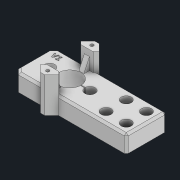
# Autodesk Inventor part: z-top
Saved by Autodesk Inventor 2021 (Build 250183000, 183)
## iProperties
Created: 2021-06-08
Part Number: z-top
Material: Generic
Document SubType Name: Modeling
Designer: arbra
Density: 1 g/cm^3
Appearance: Default
Author: arbra
Autodesk Inventor part; units mm, degrees
ref_plane "YZ Plane" through (0, 0, 0) normal (1, 0, 0) x (0, 1, 0)
ref_plane "XZ Plane" through (0, 0, 0) normal (0, 1, 0) x (-1, 0, 0)
ref_plane "XY Plane" through (0, 0, 0) normal (0, 0, 1) x (1, 0, 0)
sketch "Sketch1" plane through (0, 0, 0) normal (0, 1, 0) x (-1, 0, 0)
  line L0 (0, -40.5879) -> (0, 40.5879) construction
  line L1 (-98.4, 0) -> (58.4, 0) construction
  circle A0 centre (0, 0) radius 5
  arc A1 (14.9389, -0.375) -> (14.9389, 0.375) centre (20, 0) ccw
  line L2 (14.9389, -0.375) -> (8.9389, -0.375)
  line L3 (8.9389, -0.375) -> (8.9389, 0.375)
  line L4 (8.9389, 0.375) -> (14.9389, 0.375)
  line L5 (20, 0) -> (8.9389, 0) construction
  arc A2 (-14.9389, 0.375) -> (-14.9389, -0.375) centre (-20, 0) ccw
  line L6 (-14.9389, -0.375) -> (-8.9389, -0.375)
  line L7 (-8.9389, -0.375) -> (-8.9389, 0.375)
  line L8 (-8.9389, 0.375) -> (-14.9389, 0.375)
  line L9 (-36, 20) -> (-76, 20) construction
  line L10 (-76, 20) -> (-76, -20)
  line L11 (-76, -20) -> (-36, -20) construction
  line L12 (-36, -20) -> (-36, 20) construction
  line L13 (-36, 20) -> (-76, -20) construction
  line L14 (-76, 20) -> (-36, -20) construction
  line L15 (-46, 10) -> (-66, 10) construction
  line L16 (-66, 10) -> (-66, -10) construction
  line L17 (-66, -10) -> (-46, -10) construction
  line L18 (-46, -10) -> (-46, 10) construction
  line L19 (-46, 10) -> (-66, -10) construction
  line L20 (-66, 10) -> (-46, -10) construction
  line L21 (36, -20) -> (-76, -20)
  line L22 (-76, -20) -> (-76, 20) construction
  line L23 (-76, 20) -> (36, 20)
  line L24 (36, 20) -> (36, -20)
  line L25 (0, 21.9203) -> (-21.9203, 0) construction
  line L26 (-21.9203, 0) -> (0, -21.9203) construction
  line L27 (0, -21.9203) -> (21.9203, 0) construction
  line L28 (21.9203, 0) -> (0, 21.9203) construction
  line L29 (0, 21.9203) -> (0, -21.9203) construction
  line L30 (-21.9203, 0) -> (21.9203, 0) construction
  line L31 (0, -28.9914) -> (-28.9914, 0)
  line L32 (-28.9914, 0) -> (0, 28.9914)
  line L33 (0, 28.9914) -> (28.9914, 0)
  line L34 (28.9914, 0) -> (0, -28.9914)
  point P0 (-56, 0)
  point P1 (8.9914, 20)
  point P2 (-8.9914, 20)
  point P3 (8.9914, -20)
  point P4 (-8.9914, -20)
  dimension "d0" = 10
  dimension "d1" = 0.75
  dimension "d2" = 6
  dimension "d3" = 10.15
  dimension "d4" = 40
  dimension "d6" = 40
  dimension "d7" = 40
  dimension "d8" = 16
  dimension "d9" = 20
  dimension "d10" = 16
  dimension "d16" = 31
  dimension "d17" = 5
  constraints: 66 end point, 11 parallel, 8 midpoint, 7 perpendicular, 6 coincident, 5 collinear, 5 point on line, 5 symmetric about line, 4 point on circle, 3 centre point, 3 horizontal, 5 other
  measures "d0" diameter of A0
  measures "d1" distance of L2.end L3.end
  measures "d2" distance of L2.start L2.end
  measures "d3" diameter of A1
  measures "d4" distance of A2.centre L5.start
  measures "d6" distance of L9.end L10.end
  measures "d7" distance of L10.end L11.end
  measures "d8" distance from line of L12 A2.centre
  measures "d9" distance of L15.end L16.end
  measures "d10" distance from line of L24 L5.start
  measures "d16" distance of L25.end L26.end
  measures "d17" distance between parallel lines of L27 L34
extrude "base" add sketch "Sketch1" along normal blind 17
sketch "Sketch3" plane through (0, 17, 0) normal (0, 1, 0) x (1, 0, 0)
  circle A0 centre (0, 0) radius 11
  dimension "d18" = 22
  constraints: 1 centre point, 1 coincident
  measures "d18" diameter of A0
extrude "center hole" cut sketch "Sketch3" against normal blind 17
sketch "Sketch4" plane through (0, 17, 0) normal (0, 1, 0) x (1, 0, 0)
  line L0 (0, 28.9914) -> (-8.9914, 20) projected
  line L1 (8.9914, 20) -> (0, 28.9914) projected
  line L2 (0, 28.9914) -> (-8.9914, 20) construction
  line L3 (-8.9914, 20) -> (8.9914, 20) construction
  line L4 (-5.9914, 17) -> (-8.9914, 20)
  line L5 (8.9914, 20) -> (5.9914, 17)
  line L6 (-5.9914, 17) -> (5.9914, 17)
  line L7 (98.4, 0) -> (-58.4, 0) construction
  line L8 (0, -28.9914) -> (-8.9914, -20)
  line L9 (8.9914, -20) -> (0, -28.9914)
  line L10 (-5.9914, -17) -> (-8.9914, -20)
  line L11 (8.9914, -20) -> (5.9914, -17)
  line L12 (-5.9914, -17) -> (5.9914, -17)
  point P0 (0, 0)
  point P1 (0, 11.0086)
  dimension "d21" = 3
  constraints: 18 end point, 6 symmetric about line, 2 horizontal, 2 perpendicular
  measures "d21" distance between parallel lines of L3 L6
extrude "stepper supports" add sketch "Sketch4" along normal blind 18
hole "stepper mount" at (0, 0, -21.9203) at (0, 0, 21.9203) direction (0, 1, 0) diameter 3.2 end through all counterbore diameter 6.4 counterbore depth 22
chamfer "Chamfer2" distance 3 angle 45 2 edges at (0, 17.5, -28.9914) (0, 17.5, 28.9914)
sketch "Sketch5" plane through (0, 17, 0) normal (0, 1, 0) x (1, 0, 0)
  point P0 (0, 0)
  point P1 (46, -10)
  point P2 (66, -10)
  point P3 (66, 10)
  point P4 (46, 10)
hole "extrusion mount" at (46, 17, -10) at (66, 17, -10) at (46, 17, 10) at (66, 17, 10) direction (0, -1, 0) diameter 5.5 end through all counterbore diameter 10 counterbore depth 7
chamfer "Chamfer3" distance 5 angle 45 2 edges at (-36, 8.5, 20) (-36, 8.5, -20)
chamfer "Chamfer4" distance 2 angle 45 10 edges at (42.4957, 17, -20) (76, 17, 0) (42.4957, 17, 20) (-19.9957, 17, 20) (-33.5, 17, 17.5) (-36, 17, 0) (-33.5, 17, -17.5) (-19.9957, 17, -20) (76, 8.5, 20) (76, 8.5, -20)
sketch "Sketch6" plane through (0, 0, 0) normal (1, 0, 0) x (0, 1, 0)
  line L0 (17, -17) -> (35, -17) construction
  line L1 (17, -0.375) -> (17, -11.5) construction
  line L2 (29, -17) -> (17, -11.5)
  line L3 (-7, 0) -> (42, 0) construction
  line L4 (29, 17) -> (17, 11.5)
  point P0 (0, 0)
  dimension "d64" = 12
  dimension "d65" = 5.5
  constraints: 4 end point, 2 symmetric about line, 1 point on line
  measures "d64" horizontal distance of L2.start L1.end
  measures "d65" vertical distance of L2.start L1.end
extrude "support1" add sketch "Sketch6" along normal mid plane 5 rib yes fills toward (22.9792, -14.2955) open curves L2
extrude "support2" add sketch "Sketch6" along normal mid plane 5 rib yes fills toward (22.9792, 14.2955) open curves L4
sketch "Sketch7" plane through (0, 17, 0) normal (0, 1, 0) x (1, 0, 0)
  line L0 (-29.8273, 14.8337) -> (-25.038, 14.8337) construction
  line L1 (-25.038, 14.8337) -> (-25.038, 11.7758) construction
  line L2 (-25.038, 11.7758) -> (-29.8273, 11.7758) construction
  line L3 (-29.8273, 11.7758) -> (-29.8273, 14.8337) construction
  line L4 (-25.1353, 14.8216) -> (-26.8532, 9.8216)
  line L5 (-26.8532, 9.8216) -> (-28.162, 9.8216)
  line L6 (-28.162, 9.8216) -> (-29.88, 14.8216)
  line L7 (-29.88, 14.8216) -> (-28.5793, 14.8216)
  line L8 (-28.5793, 14.8216) -> (-27.4894, 11.4302)
  line L9 (-27.4894, 11.4302) -> (-26.4035, 14.8216)
  line L10 (-26.4035, 14.8216) -> (-25.1353, 14.8216)
  line L11 (-21.2293, 9.8216) -> (-24.5315, 9.8216)
  line L12 (-24.5315, 9.8216) -> (-24.5315, 10.6927)
  line L13 (-24.5315, 10.6927) -> (-23.478, 10.6927)
  line L14 (-23.478, 10.6927) -> (-23.478, 13.3386)
  line L15 (-23.478, 13.3386) -> (-24.5315, 13.3386)
  line L16 (-24.5315, 13.3386) -> (-24.5315, 14.153)
  spline S0 degree 2 poles (-24.5315, 14.153) (-24.3006, 14.153) (-23.8427, 14.2138) (-23.705, 14.2786) knots 0 0 0 1 2 2 2
  spline S1 degree 2 poles (-23.705, 14.2786) (-23.5469, 14.3596) (-23.3686, 14.6311) (-23.3524, 14.8337) knots 0 0 0 1 2 2 2
  line L17 (-23.3524, 14.8337) -> (-22.2584, 14.8337)
  line L18 (-22.2584, 14.8337) -> (-22.2584, 10.6927)
  line L19 (-22.2584, 10.6927) -> (-21.2293, 10.6927)
  line L20 (-21.2293, 10.6927) -> (-21.2293, 9.8216)
  point P0 (0, 0)
  constraints: 2 other
emboss "version" sketch "Sketch7" operation cut depth 0.5 direction (0, -1, 0)
equation "\"d19\" = d11"
equation "\"d11\" = 17"
body "Solid1"
